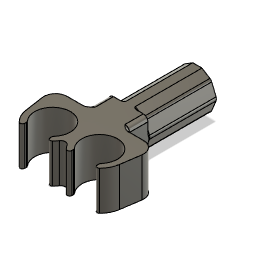
Spar_Halter v1 (Autodesk Fusion 360 design; units mm, degrees)
Autodesk Fusion 360 part; units mm, degrees
sketch "Skizze1" plane through (0, 0, 0) normal (0, 1, 0) x (1, 0, 0)
  circle A0 centre (-10.25, -10.25) radius 7.75
  circle A1 centre (10.25, -10.25) radius 7.75
  circle A2 centre (-10.25, -10.25) radius 10.25
  circle A3 centre (10.25, -10.25) radius 10.25
  line L0 (0, -10.25) -> (0, 0)
  line L1 (-10.25, 0) -> (10.25, 0)
  line L2 (-22.5, 2.5) -> (22.5, 2.5)
  line L3 (22.5, 2.5) -> (20.3894, -11.7516)
  line L4 (-22.5, 2.5) -> (-20.3894, -11.7516)
  line L5 (-15.75, -15.7101) -> (-15.75, -18.8994)
  line L6 (-4.75, -15.7101) -> (-4.75, -18.8994)
  line L7 (4.75, -15.7101) -> (4.75, -18.8994)
  line L8 (15.75, -15.7101) -> (15.75, -18.8994)
  line L9 (-15.75, -15.7101) -> (-4.75, -15.7101)
  line L10 (4.75, -15.7101) -> (15.75, -15.7101)
  dimension "d1" = 15.5
  dimension "d3" = 2.5
  dimension "d4" = 11
  dimension "d5" = 2.5
  dimension "d6" = 45
  dimension "d7" = 22.5
  constraint equal A0 A1
  constraint concentric A0 A2
  constraint concentric A1 A3
  constraint equal A2 A3
  constraint tangent A2 A3
  constraint coincident A3 L0.start
  constraint coincident A2 L0.start
  constraint tangent A2 L0
  constraint vertical L0
  constraint coincident L0.end origin
  constraint coincident A2 L1.start
  constraint coincident A3 L1.end
  constraint tangent A3 L1
  constraint tangent A2 L1
  constraint coincident L0.end L1
  constraint horizontal L2
  constraint coincident A3 L3.end
  constraint tangent A3 L3
  constraint coincident A2 L4.end
  constraint tangent A2 L4
  constraint coincident A0 L5.start
  constraint coincident A2 L5.end
  constraint parallel L0 L5
  constraint coincident A0 L6.start
  constraint coincident A2 L6.end
  constraint parallel L5 L6
  constraint coincident A1 L7.start
  constraint coincident A3 L7.end
  constraint parallel L6 L7
  constraint coincident A1 L8.start
  constraint coincident A3 L8.end
  constraint parallel L7 L8
  constraint perpendicular L6 L9
  constraint perpendicular L8 L10
  constraint equal L9 L10
  constraint collinear L9 L10
  measures "d1" diameter of A0
  measures "d3" distance of A0 A2
  measures "d4" distance of L5.start L6.start
  measures "d5" distance of L1 L2
  measures "d6" distance of L2.start L2.end
  measures "d7" horizontal distance of L0.end L2.start
extrude "Extrusion1" add sketch "Skizze1" along normal mid plane 17 contours A0 A2 L5 L6 | A2 A3 L1 L2 L3 L4 | A3 L0 L1 | A1 A3 L7 L8 | A2 L0 L1 picked at (-2.7521, -15.9178) picked at (3.6155, -16.9077) makes body 1
fillet "Abrundung1" radius 5 2 edges at (22.5, 0, -2.5) (-22.5, 0, -2.5) on bodies 1
fillet "Abrundung2" radius 2 1 edges at (0, 0, 10.25) on bodies 1
fillet "Abrundung3" radius 1 8 edges at (-15.75, 0, 18.8994) (15.75, 0, 18.8994) (4.75, 0, 18.8994) (-4.75, 0, 18.8994) (15.75, 0, 15.7101) (4.75, 0, 15.7101) (-15.75, 0, 15.7101) (-4.75, 0, 15.7101) on bodies 1
sketch "Skizze2" plane through (0, 0, -2.5) normal (0, 0, -1) x (-1, 0, 0)
  line L0 (16.705, -8.5) -> (16.705, 8.5)
  line L1 (16.705, 8.5) -> (-16.705, 8.5)
  line L2 (-16.705, 8.5) -> (-16.705, -8.5)
  line L3 (-16.705, -8.5) -> (16.705, -8.5)
  line L4 (0, 8.5) -> (-6.0104, 6.0104)
  line L5 (-6.0104, 6.0104) -> (-8.5, 0)
  line L6 (-8.5, 0) -> (-6.0104, -6.0104)
  line L7 (-6.0104, -6.0104) -> (0, -8.5)
  line L8 (0, -8.5) -> (6.0104, -6.0104)
  line L9 (6.0104, -6.0104) -> (8.5, 0)
  line L10 (8.5, 0) -> (6.0104, 6.0104)
  line L11 (6.0104, 6.0104) -> (0, 8.5)
  line L12 (-8.5, 8.5) -> (8.5, 8.5)
  line L13 (8.5, 8.5) -> (8.5, -8.5)
  line L14 (8.5, -8.5) -> (-8.5, -8.5)
  line L15 (-8.5, -8.5) -> (-8.5, 8.5)
  constraint midpoint L1 L4.start
  constraint horizontal L12
  constraint vertical L13
  constraint horizontal L14
  constraint vertical L15
  constraint coincident L3 L13.end
  constraint coincident L1 L12.start
  constraint coincident L5.end L15
  constraint coincident L9.end L13
extrude "Extrusion2" add sketch "Skizze2" along normal blind 10 separate body contours L3 L8 L9 L13 L14 | L1 L10 L11 L12 L13 | L3 L6 L7 L14 L15 | L1 L4 L5 L12 L15 makes body 2
extrude "Extrusion3" add sketch "Skizze2" along normal blind 40 contours L4 L5 L6 L7 L8 L9 L10 L11 bodies 1 2
fillet "Abrundung4" radius 2 4 edges at (-8.5, 8.5, -7.5) (8.5, 8.5, -7.5) (-8.5, -8.5, -7.5) (8.5, -8.5, -7.5) on bodies 1
fillet "Abrundung5" radius 2 6 edges at (7.9142, -7.9142, -2.5) (8.5, 0, -2.5) (7.9142, 7.9142, -2.5) (-7.9142, 7.9142, -2.5) (-8.5, 0, -2.5) (-7.9142, -7.9142, -2.5) on bodies 1
sketch "Skizze3" plane through (0, 0, -42.5) normal (0, 0, -1) x (-1, 0, 0)
  line L0 (6.0104, 6.0104) -> (0, 8.5)
  line L1 (0, 8.5) -> (-6.0104, 6.0104)
  line L2 (-6.0104, 6.0104) -> (-8.5, 0)
  line L3 (-8.5, 0) -> (-6.0104, -6.0104)
  line L4 (-6.0104, -6.0104) -> (0, -8.5)
  line L5 (0, -8.5) -> (6.0104, -6.0104)
  line L6 (6.0104, -6.0104) -> (8.5, 0)
  line L7 (8.5, 0) -> (6.0104, 6.0104)
  line L8 (0, 6.5) -> (-4.5962, 4.5962)
  line L9 (-4.5962, 4.5962) -> (-6.5, 0)
  line L10 (-6.5, 0) -> (-4.5962, -4.5962)
  line L11 (-4.5962, -4.5962) -> (0, -6.5)
  line L12 (0, -6.5) -> (4.5962, -4.5962)
  line L13 (4.5962, -4.5962) -> (6.5, 0)
  line L14 (6.5, 0) -> (4.5962, 4.5962)
  line L15 (4.5962, 4.5962) -> (0, 6.5)
  dimension "d20" = 6.5
  constraint vertical L8.start origin
  measures "d20" distance of L8.start origin
extrude "Extrusion4" cut sketch "Skizze3" against normal blind 40 contours L8 L9 L10 L11 L12 L13 L14 L15 bodies 1
sketch "Skizze4" plane through (0, 0, -42.5) normal (0, 0, -1) x (-1, 0, 0)
  line L0 (-4.5962, 4.5962) -> (0, 6.5)
  line L1 (0, 6.5) -> (4.5962, 4.5962)
  line L2 (4.5962, 4.5962) -> (6.5, 0)
  line L3 (6.5, 0) -> (4.5962, -4.5962)
  line L4 (4.5962, -4.5962) -> (0, -6.5)
  line L5 (0, -6.5) -> (-4.5962, -4.5962)
  line L6 (-4.5962, -4.5962) -> (-6.5, 0)
  line L7 (-6.5, 0) -> (-4.5962, 4.5962)
  line L8 (6.0104, 6.0104) -> (0, 8.5)
  line L9 (0, 8.5) -> (-6.0104, 6.0104)
  line L10 (-6.0104, 6.0104) -> (-8.5, 0)
  line L11 (-8.5, 0) -> (-6.0104, -6.0104)
  line L12 (-6.0104, -6.0104) -> (0, -8.5)
  line L13 (0, -8.5) -> (6.0104, -6.0104)
  line L14 (6.0104, -6.0104) -> (8.5, 0)
  line L15 (8.5, 0) -> (6.0104, 6.0104)
  line L16 (0, 8.5) -> (-2, 8.5)
  line L17 (-2, 8.5) -> (-6.0104, 6.0104)
  line L18 (0, 2.5) -> (0, 20)
  line L19 (2, 8.5) -> (6.0104, 6.0104)
  line L20 (0, 8.5) -> (2, 8.5)
  line L21 (0, 8.5) -> (6.0104, 6.0104)
  line L22 (-20, 0) -> (-2.5, 0)
  line L23 (0, -8.5) -> (-6.0104, -6.0104)
  line L24 (2, -8.5) -> (6.0104, -6.0104)
  line L25 (6.0104, -6.0104) -> (0, -8.5)
  line L26 (0, -8.5) -> (6.0104, -6.0104)
  line L27 (-2, -8.5) -> (-6.0104, -6.0104)
  line L28 (0, -8.5) -> (2, -8.5)
  line L29 (0, -8.5) -> (-2, -8.5)
  point P0 (0, 6.5)
  point P1 (0, -6.5)
  point P2 (0, -6.5)
  dimension "d23" = 2
  constraint coincident L8.end L9.start
  constraint horizontal L16
  constraint coincident L9.end L10.start
  constraint symmetric P0 L18 L0.end
  constraint symmetric L8.end L18 L9.start
  constraint symmetric L9.end L18 L8.start
  constraint symmetric L16.end L18 L19.start
  constraint symmetric P0 L22 P1
  constraint symmetric L8.start L22 L13.end
  constraint symmetric L8.end L22 L12.end
  constraint symmetric L9.end L22 L11.end
  constraint symmetric L16.end L22 L27.start
  constraint symmetric P0 L22 P2
  constraint symmetric L19.start L22 L24.start
  measures "d23" distance of L8.end L16.end
extrude "Extrusion5" add sketch "Skizze4" against normal blind 30 contours L8 L19 L20 L21 | L9 L16 L17 | L12 L23 L27 L29 | L13 L24 L25 L26 L28 bodies 1
fillet "Abrundung6" radius 2 6 edges at (-6.0104, 6.0104, -27.5) (-8.5, 0, -27.5) (-6.0104, -6.0104, -27.5) (6.0104, 6.0104, -27.5) (8.5, 0, -27.5) (6.0104, -6.0104, -27.5) on bodies 1
fillet "Abrundung7" radius 1 14 edges at (-3.7319, -7.4249, -12.5) (-5.9334, -5.9451, -12.5) (-7.2198, -3.0907, -12.5) (-8.3352, 0, -12.5) (-7.2198, 3.0907, -12.5) (-5.9334, 5.9451, -12.5) (-3.7319, 7.4249, -12.5) (3.7319, -7.4249, -12.5) (5.9334, -5.9451, -12.5) (7.2198, -3.0907, -12.5) (8.3352, 0, -12.5) (7.2198, 3.0907, -12.5) (5.9334, 5.9451, -12.5) (3.7319, 7.4249, -12.5) on bodies 1
equation "d7 = d6 / 2"
equation "d8 = ( 17 / 2 ) * 1 mm"
